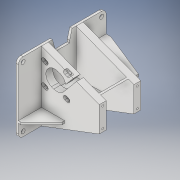
# Autodesk Inventor part: MotorSupport
Saved by Autodesk Inventor 2019.3 (Build 233278000, 278)
## iProperties
Created: 2019-06-25
Part Number: MotorSupport
Material: PC/ABS Plastic
Document SubType Name: Modeling
Designer: mark
Density: 0.357273 g/cm^3
Appearance: Smooth - White
Author: mark
Autodesk Inventor part; units mm, degrees
ref_plane "YZ Plane" through (0, 0, 0) normal (1, 0, 0) x (0, 1, 0)
ref_plane "XZ Plane" through (0, 0, 0) normal (0, 1, 0) x (-1, 0, 0)
ref_plane "XY Plane" through (0, 0, 0) normal (0, 0, 1) x (1, 0, 0)
sketch "Sketch1" plane through (0, 0, 0) normal (0, 0, 1) x (1, 0, 0)
  circle A0 centre (12.7, 19.05) radius 4 projected
  line L0 (-1.3, 46.55) -> (-1.3, -8.45)
  line L1 (-1.3, -8.45) -> (-126.3, -55.95)
  line L2 (-126.3, -55.95) -> (-126.3, 94.05)
  line L3 (-126.3, 94.05) -> (-1.3, 46.55)
  point P0 (0, 0)
  dimension "d0" = 55
  dimension "d1" = 27.5
  dimension "d2" = 14
  dimension "d3" = 150
  dimension "d4" = 125
  constraints: 8 end point, 2 vertical, 1 equal length
  measures "d0" distance of L0.end L0.start
  measures "d1" vertical distance of L0.start A0.centre
  measures "d2" distance from line of L0 A0.centre
  measures "d3" distance of L1.end L2.end
  measures "d4" distance between parallel lines of L2 L0
extrude "Extrusion1" add sketch "Sketch1" along normal blind 15 contours L0 L1 L2 L3
sketch "Sketch2" plane through (-126.3, -55.95, 0) normal (-1, 0, 0) x (0, 0, 1)
  line L0 (0, 0) -> (0, 150) projected
  line L1 (0, 0) -> (15, 0) projected
  line L2 (15, 150) -> (15, 0) projected
  line L3 (0, 150) -> (15, 150) projected
  point P0 (0, 55.95)
extrude "Extrusion2" add sketch "Sketch2" along normal blind 5
sketch "Sketch3" plane through (0, 0, 0) normal (0, 0, -1) x (-1, 0, 0)
  line L0 (1.3, 46.55) -> (1.3, -8.45) projected
  line L1 (1.3, -8.45) -> (126.3, -55.95) projected
  line L2 (126.3, -55.95) -> (131.3, -55.95) projected
  line L3 (131.3, 94.05) -> (131.3, -55.95) projected
  line L4 (126.3, 94.05) -> (131.3, 94.05) projected
  line L5 (126.3, 94.05) -> (1.3, 46.55) projected
  point P0 (0, 0)
extrude "Extrusion3" add sketch "Sketch3" along normal blind 75
sketch "Sketch4" plane through (-131.3, -55.95, 15) normal (0, -1, 0) x (1, 0, 0)
  line L0 (130, 0) -> (130, -90) projected
  line L1 (5, 0) -> (130, 0) projected
  line L2 (5, 0) -> (5, -90) projected
  line L3 (130, -90) -> (5, -90) projected
  line L4 (5, -15) -> (130, -15)
  line L5 (130, -15) -> (130, -75)
  line L6 (130, -75) -> (5, -75)
  line L7 (5, -75) -> (5, -15)
  point P0 (131.3, -15)
  dimension "d11" = 15
  dimension "d12" = 15
  constraints: 8 end point, 2 collinear
  measures "d11" distance between parallel lines of L1 L4
  measures "d12" distance between parallel lines of L3 L6
extrude "Extrusion4" cut sketch "Sketch4" against normal up to surface (150 mm away) contours L0 L6 L2 L4
sketch "Sketch5" plane through (-131.3, -55.95, 15) normal (0, -1, 0) x (1, 0, 0)
  line L0 (5, -29.125) -> (0, -29.125)
  line L1 (0, -29.125) -> (0, -60.875)
  line L2 (0, -60.875) -> (5, -60.875)
  line L3 (5, -60.875) -> (5, -29.125)
  line L4 (5, -15) -> (5, -75) projected
  line L5 (0, 0) -> (0, -90) projected
  line L6 (5, -90) -> (0, -90) projected
  point P0 (131.3, -15)
  dimension "d15" = 31.75
  dimension "d16" = 29.125
  constraints: 8 end point, 2 collinear, 1 horizontal
  measures "d15" distance of L2.end L0.start
  measures "d16" distance between parallel lines of L6 L2
extrude "Extrusion5" cut sketch "Sketch5" against normal blind 25
sketch "Sketch6" plane through (0, 0, 15) normal (0, 0, 1) x (1, 0, 0)
  line L0 (-1.3, -8.45) -> (-1.3, 46.55) projected
  line L1 (-1.3, 46.55) -> (-126.3, 94.05) projected
  line L2 (-126.3, 94.05) -> (-131.3, 94.05) projected
  line L3 (-131.3, -55.95) -> (-131.3, 94.05) projected
  line L4 (-126.3, -55.95) -> (-131.3, -55.95) projected
  line L5 (-126.3, -55.95) -> (-1.3, -8.45) projected
  line L6 (-126.3, 94.05) -> (-1.3, 46.55) projected
  line L7 (-126.3, 94.05) -> (-126.3, -55.95)
  line L8 (-126.3, 94.05) -> (-131.3, 94.05)
  line L9 (-131.3, -55.95) -> (-131.3, 94.05) projected
  line L10 (-126.3, -55.95) -> (-131.3, -55.95) projected
  line L11 (-131.3, -55.95) -> (-126.3, -55.95)
  point P0 (0, 0)
  constraints: 6 end point
extrude "Extrusion6" add sketch "Sketch6" along normal blind 50 contours L4 L3 L2 L7
sketch "Sketch7" plane through (0, 0, -75) normal (0, 0, -1) x (-1, 0, 0)
  line L0 (131.3, -55.95) -> (131.3, -30.95) projected
  line L1 (131.3, 94.05) -> (126.3, 94.05) projected
  line L2 (131.3, -55.95) -> (126.3, -55.95)
  line L3 (126.3, -55.95) -> (126.3, 94.05)
  line L4 (126.3, 94.05) -> (131.3, 94.05)
  line L5 (131.3, 94.05) -> (131.3, -55.95)
  point P0 (0, 0)
  constraints: 8 end point, 2 vertical
extrude "Extrusion7" add sketch "Sketch7" along normal blind 50
sketch "Sketch8" plane through (-126.3, -55.95, -60) normal (1, 0, 0) x (0, 0, -1)
  circle A0 centre (-115, 140) radius 4.5
  circle A1 centre (-115, 10) radius 4.5
  circle A2 centre (55, 10) radius 4.5
  circle A3 centre (55, 140) radius 4.5
  line L0 (-125, 0) -> (-125, 150) projected
  line L1 (-75, 150) -> (-125, 150) projected
  line L2 (-75, 0) -> (-125, 0) projected
  line L3 (65, 150) -> (65, 0) projected
  line L4 (15, 150) -> (65, 150) projected
  line L5 (15, 0) -> (65, 0) projected
  point P0 (-60, 55.95)
  dimension "d23" = 9
  dimension "d24" = 9
  dimension "d25" = 9
  dimension "d26" = 9
  dimension "d27" = 10
  dimension "d28" = 10
  dimension "d29" = 10
  dimension "d30" = 10
  dimension "d31" = 10
  dimension "d32" = 10
  dimension "d33" = 10
  dimension "d34" = 10
  constraints: 4 centre point
  measures "d23" diameter of A0
  measures "d24" diameter of A1
  measures "d25" diameter of A2
  measures "d26" diameter of A3
  measures "d27" distance from line of L0 A0.centre
  measures "d28" distance from line of L1 A0.centre
  measures "d29" distance from line of L2 A1.centre
  measures "d30" distance from line of L0 A1.centre
  measures "d31" distance from line of L3 A3.centre
  measures "d32" distance from line of L4 A3.centre
  measures "d33" distance from line of L3 A2.centre
  measures "d34" distance from line of L5 A2.centre
extrude "Extrusion8" cut sketch "Sketch8" against normal up to next
sketch "Sketch9" plane through (-126.3, -55.95, -60) normal (1, 0, 0) x (0, 0, -1)
  line L0 (15, 102.5) -> (65, 102.5)
  line L1 (65, 102.5) -> (65, 97.5)
  line L2 (65, 97.5) -> (15, 97.5)
  line L3 (15, 97.5) -> (15, 102.5)
  line L4 (15, 52.5) -> (65, 52.5)
  line L5 (65, 52.5) -> (65, 47.5)
  line L6 (65, 47.5) -> (15, 47.5)
  line L7 (15, 47.5) -> (15, 52.5)
  line L8 (15, 150) -> (15, 102.5) projected
  line L9 (15, 102.5) -> (15, 47.5) projected
  line L10 (65, 150) -> (65, 0) projected
  line L11 (15, 150) -> (65, 150) projected
  line L12 (15, 102.5) -> (0, 102.5) projected
  line L13 (0, 47.5) -> (15, 47.5) projected
  point P0 (40, 97.5)
  dimension "d77" = 5
  constraints: 16 end point, 7 collinear, 4 horizontal, 1 midpoint
  measures "d77" distance of L0.end L1.end
extrude "Extrusion9" add sketch "Sketch9" along normal blind 110 contours L0 L1 L2 L3 | L4 L5 L6 L7
chamfer "Chamfer3" distance 40 distance2 100 1 edges at (-16.3, -5.95, -125) measured on face at (-16.3, -5.95, -124.5)
chamfer "Chamfer4" distance 40 distance2 100 1 edges at (-16.3, 44.05, -125) measured on face at (-16.3, 44.05, -124.5)
fillet "Fillet1" radius 10 4 edges at (-128.8, 94.05, 65) (-128.8, -55.95, 65) (-128.8, -55.95, -125) (-128.8, 94.05, -125)
chamfer "Chamfer5" distance 20 angle 15 1 edges at (-128.8, -55.95, -45.875) measured on face at (-128.8, -55.45, -45.875)
chamfer "Chamfer6" distance 20 angle 15 1 edges at (-128.8, -55.95, -14.125) measured on face at (-128.8, -55.45, -14.125)
sketch "Sketch10" plane through (-1.3, -8.45, 15) normal (1, 0, 0) x (0, 0, -1)
  circle A0 centre (7.5, 48.75) radius 2
  circle A1 centre (7.5, 6.25) radius 2
  circle A2 centre (82.5, 6.25) radius 2
  circle A3 centre (82.5, 48.75) radius 2
  line L0 (15, 0) -> (15, 55) projected
  line L1 (90, 55) -> (90, 0) projected
  line L2 (0, 0) -> (0, 55) projected
  line L3 (90, 55) -> (75, 55) projected
  line L4 (15, 55) -> (0, 55) projected
  point P0 (15, 8.45)
  dimension "d61" = 7.5
  dimension "d62" = 7.5
  dimension "d63" = 7.5
  dimension "d64" = 7.5
  dimension "d65" = 42.5
  dimension "d66" = 42.5
  dimension "d67" = 6.25
  dimension "d68" = 6.25
  dimension "d69" = 4
  dimension "d70" = 4
  dimension "d71" = 4
  dimension "d72" = 4
  constraints: 4 centre point
  measures "d61" distance from line of L0 A0.centre
  measures "d62" distance from line of L1 A3.centre
  measures "d63" distance from line of L1 A2.centre
  measures "d64" distance from line of L2 A1.centre
  measures "d65" distance of A1.centre A0.centre
  measures "d66" distance of A2.centre A3.centre
  measures "d67" distance from line of A3.centre L3
  measures "d68" distance from line of L4 A0.centre
  measures "d69" diameter of A0
  measures "d70" diameter of A1
  measures "d71" diameter of A3
  measures "d72" diameter of A2
extrude "Extrusion10" cut sketch "Sketch10" against normal blind 25
sketch "Sketch11" plane through (0, 0, 15) normal (0, 0, 1) x (1, 0, 0)
  circle A0 centre (-97.8, 46.4143) radius 19.05
  circle A1 centre (-74.23, 22.8443) radius 2.6
  arc A2 (-73.3064, 72.4148) -> (-75.1536, 67.5539) centre (-74.23, 69.9843) ccw
  circle A3 centre (-121.37, 69.9843) radius 2.6
  circle A4 centre (-121.37, 22.8443) radius 2.6
  line L0 (-126.3, 94.05) -> (-126.3, -55.95) projected
  line L1 (-74.23, 69.9843) -> (-121.37, 69.9843)
  line L2 (-1.3, 46.55) -> (-126.3, 94.05) projected
  circle A5 centre (-92.8, 44.5143) radius 19.05
  circle A6 centre (-69.23, 20.9443) radius 2.6
  arc A7 (-70.1536, 65.6539) -> (-68.3064, 70.5148) centre (-69.23, 68.0843) ccw
  circle A8 centre (-116.37, 68.0843) radius 2.6
  circle A9 centre (-116.37, 20.9443) radius 2.6
  line L3 (-69.23, 68.0843) -> (-116.37, 68.0843)
  line L4 (-73.3064, 72.4148) -> (-68.3064, 70.5148)
  line L5 (-70.1536, 65.6539) -> (-75.1536, 67.5539)
  line L6 (-86.0331, 62.322) -> (-91.0331, 64.222)
  line L7 (-99.5669, 26.7067) -> (-104.5669, 28.6067)
  line L8 (-115.4464, 70.5148) -> (-120.4464, 72.4148)
  line L9 (-117.2936, 65.6539) -> (-122.2936, 67.5539)
  line L10 (-115.4464, 23.3748) -> (-120.4464, 25.2748)
  line L11 (-117.2936, 18.5139) -> (-122.2936, 20.4139)
  line L12 (-68.3064, 23.3748) -> (-73.3064, 25.2748)
  line L13 (-70.1536, 18.5139) -> (-75.1536, 20.4139)
  line L14 (-1.3, 46.55) -> (-1.3, -8.45) projected
  line L15 (-126.3, 94.05) -> (-1.3, 46.55) projected
  line L16 (-50.5273, 65.2564) -> (-78.2069, 32.2692)
  line L17 (-57.456, 67.8893) -> (-74.0851, 48.0715)
  line L18 (-50.5273, 65.2564) -> (-57.456, 67.8893)
  point P0 (0, 0)
  point P1 (-81.37, 76.9766)
  point P2 (-81.37, 59.7543)
  point P3 (-75.6243, 52.7543)
  dimension "d79" = 5.2
  dimension "d80" = 5.2
  dimension "d81" = 5.2
  dimension "d82" = 38.1
  dimension "d83" = 47.14
  dimension "d84" = 47.14
  dimension "d85" = 47.14
  dimension "d86" = 47.14
  dimension "d87" = 23.57
  dimension "d88" = 23.57
  dimension "d89" = 4.93
  dimension "d90" = 4.93
  dimension "d91" = 4
  dimension "d94" = 5.2
  dimension "d95" = 5.2
  dimension "d96" = 5.2
  dimension "d97" = 5.2
  dimension "d98" = 38.1
  dimension "d99" = 47.14
  dimension "d100" = 47.14
  dimension "d101" = 47.14
  dimension "d102" = 47.14
  dimension "d103" = 23.57
  dimension "d104" = 23.57
  dimension "d105" = 4
  dimension "d106" = 5
  dimension "d107" = 5
  dimension "d124" = 2.6
  dimension "d126" = 7
  dimension "d127" = 40
  dimension "d128" = 7
  constraints: 30 end point, 24 point on circle, 21 tangent, 10 centre point, 3 point on line, 2 horizontal, 1 parallel
  measures "d79" diameter of A1
  measures "d80" diameter of A3
  measures "d81" diameter of A4
  measures "d82" diameter of A0
  measures "d83" distance of L1.start A1.centre
  measures "d84" distance of A4.centre A1.centre
  measures "d85" distance of A4.centre L1.end
  measures "d86" distance of L1.end L1.start
  measures "d87" horizontal distance of A0.centre L1.start
  measures "d88" horizontal distance of A0.centre L1.start
  measures "d89" distance from line of L0 L1.end
  measures "d90" distance from line of L0 A4.centre
  measures "d91" distance from line of L1.start L2
  measures "d94" diameter of A7
  measures "d95" diameter of A6
  measures "d96" diameter of A8
  measures "d97" diameter of A9
  measures "d98" diameter of A5
  measures "d99" distance of L3.start A6.centre
  measures "d100" distance of A9.centre A6.centre
  measures "d101" distance of A9.centre L3.end
  measures "d102" distance of L3.end L3.start
  measures "d103" horizontal distance of A5.centre L3.start
  measures "d104" horizontal distance of A5.centre L3.start
  measures "d105" distance from line of L2 L3.start
  measures "d106" horizontal distance of L1.start L3.start
  measures "d107" horizontal distance of A1.centre A6.centre
  measures "d124" radius of A2
  measures "d126" vertical distance of point (-75.624, 52.754) point (-81.37, 59.754)
  measures "d127" angle of L16 L0
  measures "d128" distance between parallel lines of L17 L16
extrude "Extrusion11" cut sketch "Sketch11" against normal up to next contours A0 A5 | L6 A5 A0 | A0 A5 L7 | A5 A0 | A0 A5 | L17 L2 L16 A5 | A1 | A1 L12 A6 L13 | A6 | L4 A7 L5 A2 | A8 L1 | L1 A8 | A8 L9 A3 L1 | L1 A3 L8 A8 | A3 | A4 | A4 L10 A9 L11 | A9
sketch "Sketch12" plane through (-126.3, 94.05, 0) normal (0, 1, 0) x (1, 0, 0)
  line L0 (0, 45.875) -> (-5, 45.875)
  line L1 (-5, 45.875) -> (-5, 14.125)
  line L2 (-5, 14.125) -> (0, 14.125)
  line L3 (0, 14.125) -> (0, 45.875)
  line L4 (0, -15) -> (0, -75)
  line L5 (-5, 0) -> (-5, -15)
  line L6 (5, -15) -> (-5, -15)
  line L7 (-5, 115) -> (-5, -55) projected
  line L8 (0, 60) -> (0, 0) projected
  line L9 (125, -15) -> (0, -15) projected
  point P0 (126.3, 0)
  point P1 (131.3, -15)
  point P2 (39.1779, -15)
  dimension "d110" = 31.75
  dimension "d111" = 29.125
  constraints: 14 end point, 5 collinear, 1 horizontal
  measures "d110" distance of L2.end L0.start
  measures "d111" distance between parallel lines of L6 L2
extrude "Extrusion12" cut sketch "Sketch12" against normal blind 25
chamfer "Chamfer7" distance 20 angle 15 1 edges at (-128.8, 94.05, -45.875) measured on face at (-128.8, 93.55, -45.875)
chamfer "Chamfer8" distance 20 angle 15 1 edges at (-128.8, 94.05, -14.125) measured on face at (-128.8, 93.55, -14.125)
sketch "Sketch13" plane through (-126.3, -55.95, 0) normal (1, 0, 0) x (0, 0, -1)
  line L0 (60, 49.2943) -> (0, 49.2943)
  line L1 (0, 49.2943) -> (0, 54.2943)
  line L2 (0, 54.2943) -> (60, 54.2943)
  line L3 (60, 54.2943) -> (60, 49.2943)
  line L4 (60, 47.5) -> (60, 0) projected
  line L5 (0, 0) -> (0, 47.5) projected
  line L6 (0, 79.3248) -> (0, 74.2943) projected
  point P0 (0, 55.95)
  point P1 (0, 74.4639)
  dimension "d120" = 5
  dimension "d121" = 20
  constraints: 8 end point, 2 collinear, 1 horizontal
  measures "d120" distance between parallel lines of L2 L0
  measures "d121" distance from line of L2 L6.end
extrude "Extrusion13" add sketch "Sketch13" along normal blind 55
sketch "Sketch15" plane through (0, 0, 15) normal (0, 0, 1) x (1, 0, 0)
  arc A0 (-73.3064, 72.4148) -> (-75.1536, 67.5539) centre (-74.23, 69.9843) ccw projected
  line L0 (-70.1536, 65.6539) -> (-75.1536, 67.5539) projected
  line L1 (-73.3064, 72.4148) -> (-68.3064, 70.5148) projected
  arc A1 (-70.1536, 65.6539) -> (-68.3064, 70.5148) centre (-69.23, 68.0843) ccw projected
  arc A2 (-73.3064, 25.2748) -> (-75.1536, 20.4139) centre (-74.23, 22.8443) ccw projected
  line L2 (-73.3064, 25.2748) -> (-68.3064, 23.3748) projected
  arc A3 (-70.1536, 18.5139) -> (-68.3064, 23.3748) centre (-69.23, 20.9443) ccw projected
  line L3 (-70.1536, 18.5139) -> (-75.1536, 20.4139) projected
  arc A4 (-117.2936, 18.5139) -> (-115.4464, 23.3748) centre (-116.37, 20.9443) ccw projected
  line L4 (-120.4464, 25.2748) -> (-115.4464, 23.3748) projected
  arc A5 (-120.4464, 25.2748) -> (-122.2936, 20.4139) centre (-121.37, 22.8443) ccw projected
  line L5 (-117.2936, 18.5139) -> (-122.2936, 20.4139) projected
  arc A6 (-117.2936, 65.6539) -> (-115.4464, 70.5148) centre (-116.37, 68.0843) ccw projected
  line L6 (-117.2936, 65.6539) -> (-122.2936, 67.5539) projected
  arc A7 (-120.4464, 72.4148) -> (-122.2936, 67.5539) centre (-121.37, 69.9843) ccw projected
  line L7 (-120.4464, 72.4148) -> (-115.4464, 70.5148) projected
  arc A8 (-117.9685, 63.8778) -> (-114.7715, 72.2909) centre (-116.37, 68.0843) ccw
  line L8 (-117.9685, 63.8778) -> (-122.9685, 65.7778)
  arc A9 (-119.7715, 74.1909) -> (-122.9685, 65.7778) centre (-121.37, 69.9843) ccw
  line L9 (-119.7715, 74.1909) -> (-114.7715, 72.2909)
  arc A10 (-117.9685, 16.7378) -> (-114.7715, 25.1509) centre (-116.37, 20.9443) ccw
  line L10 (-117.9685, 16.7378) -> (-122.9685, 18.6378)
  arc A11 (-119.7715, 27.0509) -> (-122.9685, 18.6378) centre (-121.37, 22.8443) ccw
  line L11 (-119.7715, 27.0509) -> (-114.7715, 25.1509)
  arc A12 (-72.6315, 27.0509) -> (-75.8285, 18.6378) centre (-74.23, 22.8443) ccw
  line L12 (-72.6315, 27.0509) -> (-67.6315, 25.1509)
  arc A13 (-70.8285, 16.7378) -> (-67.6315, 25.1509) centre (-69.23, 20.9443) ccw
  line L13 (-70.8285, 16.7378) -> (-75.8285, 18.6378)
  arc A14 (-70.8285, 63.8778) -> (-65.7828, 65.1918) centre (-69.23, 68.0843) ccw
  line L14 (-70.8285, 63.8778) -> (-75.8285, 65.7778)
  line L15 (-126.3, 94.05) -> (-1.3, 46.55) projected
  line L16 (-77.6772, 72.8769) -> (-75.9616, 74.9214)
  line L17 (-57.456, 67.8893) -> (-126.3, 94.05) projected
  line L18 (-74.0851, 48.0715) -> (-57.456, 67.8893) projected
  line L19 (-62.0534, 69.6363) -> (-65.7828, 65.1918)
  line L20 (-62.0534, 69.6363) -> (-75.9616, 74.9214)
  arc A15 (-77.6772, 72.8769) -> (-75.8285, 65.7778) centre (-74.23, 69.9843) ccw
  point P0 (0, 0)
  dimension "d131" = 4.5
  dimension "d132" = 4.5
  dimension "d133" = 4.5
  dimension "d134" = 4.5
  dimension "d135" = 4.5
  dimension "d136" = 5
  constraints: 20 end point, 16 point on circle, 8 centre point, 3 tangent, 2 parallel, 2 point on line, 9 other
  measures "d131" radius of A14
  measures "d132" radius of A13
  measures "d133" radius of A8
  measures "d134" radius of A10
  measures "d135" radius of A15
  measures "d136" horizontal distance of L14.start L14.end
extrude "Extrusion14" cut sketch "Sketch15" against normal blind 6
sketch "Sketch16" plane through (-1.3, -8.45, 0) normal (0, 0, -1) x (-1, 0, 0)
  line L0 (70, 1.7943) -> (70, 6.7943) projected
  line L1 (70, 6.7943) -> (15.793, 61.0013)
  line L2 (0, 55) -> (49.2273, 73.7064) projected
  line L3 (70, 1.7943) -> (12.1698, 59.6245)
  line L4 (12.1698, 59.6245) -> (15.793, 61.0013)
  line L5 (0, 0) -> (0, 55) projected
  point P0 (-1.3, 8.45)
  dimension "d139" = 45
  constraints: 6 end point, 2 point on line, 1 parallel
  measures "d139" angle of L3 L5
extrude "Extrusion15" add sketch "Sketch16" along normal up to next
sketch "Sketch17" plane through (-126.3, -55.95, 15) normal (1, 0, 0) x (0, 0, -1)
  line L0 (0, 30) -> (-50, 30)
  line L1 (-50, 30) -> (-50, 35)
  line L2 (-50, 35) -> (0, 35)
  line L3 (0, 35) -> (0, 30)
  line L4 (-50, 10) -> (-50, 140) projected
  line L5 (0, 0) -> (0, 47.5) projected
  line L6 (140, 97.5) -> (140, 102.5) projected
  line L7 (0, 0) -> (-40, 0) projected
  point P0 (15, 55.95)
  dimension "d142" = 30
  constraints: 8 end point, 2 collinear, 2 parallel
  measures "d142" distance between parallel lines of L0 L7
extrude "Extrusion16" add sketch "Sketch17" along normal blind 50
chamfer "Chamfer9" distance 45 angle 45 1 edges at (-76.3, -23.45, 65)
body "Solid1"
